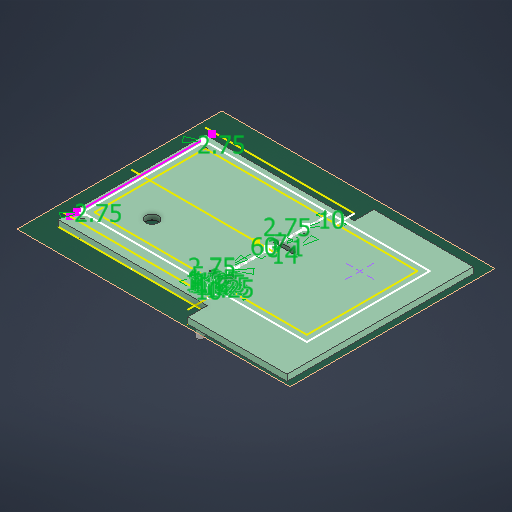
# Autodesk Inventor part: top-buggy-body-assembly-ready-group2
Saved by Autodesk Inventor 2026.2 (Build 302298010, 298A)
## iProperties
Created: 2026-02-09
Part Number: top-buggy-body-assembly-ready-group2
Material: Generic
Document SubType Name: Modeling
Designer: dm2166
Density: 1 g/cm^3
Appearance: Default
Mass: 226.605 g
Surface Area: 796.438 cm^2
Volume: 226.605 cm^3
Author: dm2166
Autodesk Inventor part; units mm, degrees
ref_plane "YZ Plane" through (0, 0, 0) normal (1, 0, 0) x (0, 1, 0)
ref_plane "XZ Plane" through (0, 0, 0) normal (0, 1, 0) x (-1, 0, 0)
ref_plane "XY Plane" through (0, 0, 0) normal (0, 0, 1) x (1, 0, 0)
sketch "Sketch1" plane through (0, 0, 0) normal (0, 1, 0) x (-1, 0, 0)
  line L0 (-85.5, -44.5) -> (85.5, -44.5)
  line L1 (85.5, -44.5) -> (85.5, 44.5)
  line L2 (85.5, 44.5) -> (-85.5, 44.5)
  line L3 (-85.5, 44.5) -> (-85.5, -44.5)
  line L4 (-85.5, -44.5) -> (85.5, 44.5) construction
  line L5 (85.5, -44.5) -> (-85.5, 44.5) construction
  line L6 (-81, -38.5) -> (81, -38.5)
  line L7 (81, -38.5) -> (81, 38.5)
  line L8 (81, 38.5) -> (-81, 38.5)
  line L9 (-81, 38.5) -> (-81, -38.5)
  line L10 (-81, -38.5) -> (81, 38.5) construction
  line L11 (81, -38.5) -> (-81, 38.5) construction
  line L12 (81, 38.5) -> (79.55, 38.5)
  line L13 (81, 37.05) -> (81, 38.5)
  circle A0 centre (79.55, 36.5) radius 1.45
  circle A1 centre (79.55, -36.5) radius 1.45
  circle A2 centre (-79.55, -38.5) radius 1.45
  circle A3 centre (-79.55, 38.4727) radius 1.45
  line L14 (81, -38.5) -> (81, -35.6)
  line L15 (-81, -38.5) -> (-78.1, -38.5)
  line L16 (-81, 38.5) -> (-81, 35.6)
  circle A4 centre (-79.55, 38.4727) radius 2.5
  line L17 (-95.5566, 0) -> (75.4434, 0)
  line L18 (0, 31.9167) -> (0, -57.0833)
  circle A5 centre (-79.55, -38.5) radius 2.5
  circle A6 centre (79.55, 36.5) radius 2.5
  circle A7 centre (79.55, -36.5) radius 2.5
  line L19 (140, 0) -> (-140, 0) projected
  line L20 (0, -105) -> (0, 105) projected
  line L21 (-100, 59.2475) -> (100, 59.2475)
  line L22 (100, 59.2475) -> (100, -59.2475)
  line L23 (100, -59.2475) -> (-100, -59.2475)
  line L24 (-100, -59.2475) -> (-100, 59.2475)
  line L25 (-100, 59.2475) -> (100, -59.2475) construction
  line L26 (100, 59.2475) -> (-100, -59.2475) construction
  line L27 (-100, 75) -> (-20, 75)
  line L28 (-20, 75) -> (-20, -75)
  line L29 (-20, -75) -> (-100, -75)
  line L30 (-100, -75) -> (-100, 75)
  line L31 (-100, 75) -> (-20, -75) construction
  line L32 (-20, 75) -> (-100, -75) construction
  line L33 (-79.55, 38.5) -> (-79.55, -38.5)
  line L34 (79.55, 36.5) -> (79.55, -36.5)
  line L35 (-96.0841, 75) -> (-26.0841, 75)
  line L36 (-26.0841, -75) -> (-94.0841, -75)
  point P0 (0, 0)
  point P1 (-80.9997, 38.5)
  point P2 (-81, 38.4727)
  point P3 (-81, -38.5)
  point P4 (-81, -38.5)
  point P5 (79.55, -38.5)
  point P6 (81, -36.5)
  point P7 (81, 36.5)
  point P8 (-60, 0)
  point P9 (-20, 59.2475)
  point P10 (-20, -59.2475)
  point P11 (-79.55, 0)
  point P12 (-78.1003, 38.5)
  point P13 (79.55, 0)
  dimension "d0" = 171
  dimension "d1" = 89
  dimension "d2" = 162
  dimension "d3" = 77
  dimension "d7" = 2.9
  dimension "d8" = 2.9
  dimension "d9" = 2.9
  dimension "d10" = 2.9
  dimension "d53" = 5
  dimension "d56" = 200
  dimension "d57" = 80
  dimension "d58" = 150
  dimension "d82" = 77
  dimension "d84" = 36.5
  dimension "d85" = 36.5
  constraints: 70 end point, 11 parallel, 10 midpoint, 8 centre point, 7 horizontal, 6 perpendicular, 5 point on line, 3 collinear, 3 concentric, 1 vertical, 4 other
  measures "d0" distance of L2.end L1.end
  measures "d1" distance of L1.end L0.end
  measures "d2" distance of L8.end L7.end
  measures "d3" distance of L7.end L6.end
  measures "d7" diameter of A0
  measures "d8" diameter of A1
  measures "d9" diameter of A2
  measures "d10" diameter of A3
  measures "d53" diameter of A4
  measures "d56" distance of L22.end L23.end
  measures "d57" distance of L28.end L29.end
  measures "d58" distance of L27.end L28.end
  measures "d82" distance of L33.start L33.end
  measures "d84" distance of point (79.55, 0) A1.centre
  measures "d85" distance from line of L19 A0.centre
extrude "Extrusion1" add sketch "Sketch1" along normal blind 55 contours A2 L6 | L6 L33 A2 | L8 L33 A3 | A3 L8 | A2 L33 L6 | L33 L8 A3 | A1 | A0
extrude "Extrusion2" add sketch "Sketch1" along normal blind 10 contours L28 L17 L18 L6 | L6 A5 L33 L17 L28 | L17 L33 A5 L9 | L9 A4 L33 L17 | L18 L17 L19 L34 A7 L6 | L6 A2 L33 A5 | L28 L8 L20 L18 L17 | L17 L33 A4 L8 L28 | A5 L33 A2 L9 | A7 L34 A1 L7 L6 | L18 L20 L8 A6 L34 L19 L17 | L6 L33 A2 | L8 L33 A3 | L9 A3 L33 A4 | A2 L33 L6 | L33 A3 L8 A4 | L19 L34 A6 L7 | L7 A7 L34 L19 | A7 L7 A1 L34 | L33 L8 A3 | A6 L34 A0 L7 | A1 | L8 L7 A0 L34 A6 | A0
extrude "Extrusion3" add sketch "Sketch1" along normal blind 25 contours L3 L17 L9 A5 L6 L28 L0 | L28 L6 L18 L0 | L3 L2 L28 L8 A4 L9 L17 | L18 L6 A7 L7 L19 L1 L0 | A5 L9 A2 L6 | L2 L20 L8 L28 | L19 L7 A6 L8 L20 L2 L1 | L6 L7 A7 | A2 L6 | A4 L8 A3 L9 | A3 L8 | L7 L8 A6
chamfer "Chamfer1" distance 2 angle 45 4 edges at (0, 25, 44.5) (85.5, 25, 0) (0, 25, -44.5) (-85.5, 25, 0)
extrude "Extrusion11" add sketch "Sketch1" along normal blind 45 contours A5 L9 A2 L6 | L6 A2 L33 A5 | A5 L33 A2 L9 | A7 L34 A1 L7 L6 | L6 L7 A7 | A2 L6 | L6 L33 A2 | L8 L33 A3 | A4 L8 A3 L9 | A3 L8 | L9 A3 L33 A4 | A2 L33 L6 | L33 A3 L8 A4 | A7 L7 A1 L34 | L33 L8 A3 | A6 L34 A0 L7 | L7 L8 A6 | A1 | L8 L7 A0 L34 A6 | A0
extrude "Extrusion12" add sketch "Sketch1" along normal blind 10 contours L0 L28 L23 L24 L19 L17 L3 | L0 L18 L20 L23 L28 | L17 L19 L24 L21 L28 L2 L3 | L0 L1 L19 L22 L23 L20 L18 | L28 L29 L30 L23 | L28 L21 L20 L2 | L1 L2 L20 L21 L22 L19 | L21 L30 L27 L28
chamfer "Chamfer2" distance 2 angle 45 8 edges at (100, 10, 0) (60, 10, 75) (20, 10, 67.1238) (60, 10, -75) (20, 10, -67.1238) (-40, 10, -59.2475) (-40, 10, 59.2475) (-100, 10, 0)
sketch "Sketch4" plane through (0, 0, 0) normal (0, -1, 0) x (1, 0, 0)
  circle A0 centre (-11.2675, 0) radius 2 projected
  circle A1 centre (-71.2675, 0) radius 2 projected
  circle A2 centre (-41.2675, 30) radius 2 projected
  circle A3 centre (-11.2675, 0) radius 2.5
  circle A4 centre (-71.2675, 0) radius 2.5
  circle A5 centre (-41.2675, 30) radius 2.5
  point P0 (0, 0)
  dimension "d64" = 5
  constraints: 3 centre point, 3 coincident, 2 equal radius
  measures "d64" diameter of A5
extrude "Extrusion13" add sketch "Sketch4" along normal blind 10 contours A0 | A1 | A2 | A3 | A4 | A5
sketch "Sketch7" plane through (0, 0, 0) normal (0, -1, 0) x (1, 0, 0)
  line L0 (20, -59.2475) -> (-100, -59.2475) projected
  line L1 (20, -75) -> (20, -59.2475) projected
  line L2 (100, -75) -> (20, -75) projected
  line L3 (100, 75) -> (100, -75) projected
  line L4 (20, 75) -> (100, 75) projected
  line L5 (20, 59.2475) -> (20, 75) projected
  line L6 (-100, 59.2475) -> (20, 59.2475) projected
  line L7 (-100, -59.2475) -> (-100, 59.2475) projected
  line L8 (-95, -54.2475) -> (25, -54.2475)
  line L9 (25, -54.2475) -> (25, -70)
  line L10 (25, -70) -> (95, -70)
  line L11 (95, -70) -> (95, 70)
  line L12 (95, 70) -> (25, 70)
  line L13 (25, 70) -> (25, 54.2475)
  line L14 (25, 54.2475) -> (-95, 54.2475)
  line L15 (-95, 54.2475) -> (-95, -54.2475)
  line L16 (-90, -49.2475) -> (30, -49.2475)
  line L17 (30, -49.2475) -> (30, -65)
  line L18 (30, -65) -> (90, -65)
  line L19 (90, -65) -> (90, 65)
  line L20 (90, 65) -> (30, 65)
  line L21 (30, 65) -> (30, 49.2475)
  line L22 (30, 49.2475) -> (-90, 49.2475)
  line L23 (-90, 49.2475) -> (-90, -49.2475)
  circle A0 centre (25, -70) radius 2.5
  circle A1 centre (25, 70) radius 2.5
  circle A2 centre (-41.2675, 0) radius 44 projected
  line L24 (-41.2675, -59.2475) -> (-41.2675, 59.2475)
  line L25 (17.4651, 0) -> (-100, 0)
  point P0 (0, 0)
  dimension "d86" = 5
  dimension "d87" = 10
  dimension "d88" = 5
  dimension "d89" = 5
  constraints: 36 end point, 3 midpoint, 2 centre point, 2 coincident, 1 perpendicular, 1 point on line, 14 other
  measures "d86" distance between parallel lines of L0 L8
  measures "d87" distance between parallel lines of L0 L16
  measures "d88" diameter of A0
  measures "d89" diameter of A1
extrude "Extrusion15" add sketch "Sketch7" along normal blind 10 contours A0 L10 L9 | L9 L10 A0 | A1 L12 L13 | L13 L12 A1
fillet "Fillet16" radius 1 1 edges at (22.5, -10, -70)
fillet "Fillet17" radius 1 1 edges at (22.5, 0, -70)
fillet "Fillet18" radius 1 1 edges at (22.5, 0, 70)
fillet "Fillet19" radius 1 1 edges at (22.5, -10, 70)
sketch "Sketch9" plane through (0, 0, 0) normal (0, -1, 0) x (1, 0, 0)
  line L0 (-100, 59.2475) -> (20, 59.2475) projected
  line L1 (20, -75) -> (20, 75) projected
  line L2 (20, -59.2475) -> (-100, -59.2475) projected
  line L3 (-100, -59.2475) -> (-100, 59.2475) projected
  circle A0 centre (-41.2675, 0) radius 44 projected
  line L4 (-41.2675, -59.2475) -> (-41.2675, 59.2475)
  line L5 (17.4651, 0) -> (-100, 0)
  line L6 (20, -54.2475) -> (-95, -54.2475)
  line L7 (-95, -54.2475) -> (-95, 54.2475)
  line L8 (-95, 54.2475) -> (20, 54.2475)
  line L9 (-41.2675, 50.5475) -> (-41.2675, 47.5475)
  point P0 (0, 0)
  point P1 (-41.2675, -54.2475)
  point P2 (-41.2675, 54.2475)
  constraints: 12 end point, 4 point on line, 3 midpoint, 1 perpendicular, 1 symmetric about line, 2 other
sketch "Sketch11" plane through (0, 10, 0) normal (0, 1, 0) x (1, 0, 0)
  circle A0 centre (-168.2379, -151.522) radius 7.5
  circle A1 centre (-62.4807, -21.2132) radius 7.5 projected
  circle A2 centre (-62.4807, -21.2132) radius 5
  point P0 (0, 0)
  dimension "d134" = 10
  constraints: 2 centre point, 1 coincident
  measures "d134" diameter of A2
sketch "Sketch12" plane through (0, 10, 0) normal (0, 1, 0) x (1, 0, 0)
  line L0 (-85.5, -44.5) -> (85.5, -44.5) projected
  line L1 (-85.5, 44.5) -> (-85.5, -44.5) projected
  line L2 (85.5, 44.5) -> (-85.5, 44.5) projected
  line L3 (85.5, -44.5) -> (85.5, 44.5) projected
  line L4 (90.5, -49.5) -> (-90.5, -49.5)
  line L5 (-90.5, -49.5) -> (-90.5, 49.5)
  line L6 (-90.5, 49.5) -> (90.5, 49.5)
  line L7 (90.5, 49.5) -> (90.5, -49.5)
  circle A0 centre (-90.5, 49.5) radius 1.375
  circle A1 centre (-90.5, -49.5) radius 1.375
  line L8 (20, -59.2475) -> (20, -75) projected
  line L9 (20, -59.2475) -> (20, -44.5)
  line L10 (20, 59.2475) -> (-100, 59.2475) projected
  line L11 (20, 59.2475) -> (20, 44.5)
  line L12 (20, -49.5) -> (10, -49.5)
  line L13 (20, 49.5) -> (10, 49.5)
  line L14 (17.4651, 0) -> (-100, 0) projected
  line L15 (10, 49.5) -> (10, -49.5)
  line L16 (10, 30) -> (10, -30)
  circle A2 centre (10, -30) radius 1.375
  circle A3 centre (10, 30) radius 1.375
  point P0 (0, 0)
  point P1 (62.481, 21.213)
  point P2 (10, 0)
  dimension "d120" = 5
  dimension "d123" = 2.75
  dimension "d124" = 2.75
  dimension "d127" = 10
  dimension "d128" = 10
  dimension "d162" = 60
  dimension "d163" = 2.75
  dimension "d164" = 2.75
  constraints: 20 end point, 10 point on line, 6 coincident, 4 centre point, 2 midpoint, 1 perpendicular, 3 other
  measures "d120" distance between parallel lines of L0 L4
  measures "d123" diameter of A0
  measures "d124" diameter of A1
  measures "d127" distance of L12.start L12.end
  measures "d128" distance of L13.start L13.end
  measures "d162" distance of L16.start L16.end
  measures "d163" diameter of A2
  measures "d164" diameter of A3
extrude "Extrusion19" cut sketch "Sketch12" against normal blind 14 contours A1 L5 L4 | L4 L5 A1 | A0 L6 L5 | L5 L6 A0
extrude "Extrusion20" [suppressed]
fillet "Fillet21" radius 1 6 edges at (-73.7675, 0, 0) (-73.7675, -10, 0) (-43.7675, -10, 30) (-43.7675, 0, 30) (-13.7675, 0, 0) (-13.7675, -10, 0)
extrude "Extrusion21" cut sketch "Sketch11" against normal blind 14 contours A2
fillet "Fillet22" radius 1 2 edges at (-67.4807, 0, 21.2132) (-67.4807, 10, 21.2132)
sketch "Sketch13" plane through (0, 0, 0) normal (0, -1, 0) x (1, 0, 0)
  line L0 (-95, 54.2475) -> (20, 54.2475) projected
  line L1 (6.8242, 54.2475) -> (3.8242, 54.2475)
  point P0 (0, 0)
  point P1 (11.8242, 54.2475)
  point P2 (-21.0705, 54.2475)
  constraints: 3 point on line, 2 end point
sketch "Sketch14" plane through (0, 10, 0) normal (0, 1, 0) x (1, 0, 0)
  line L0 (-98, 57.2475) -> (22, 57.2475) projected
  line L1 (-98, -57.2475) -> (-98, 57.2475) projected
  line L2 (22, -57.2475) -> (-98, -57.2475) projected
  line L3 (-85.5, -44.5) -> (85.5, -44.5) projected
  line L4 (-85.5, 44.5) -> (-85.5, -44.5) projected
  line L5 (85.5, 44.5) -> (-85.5, 44.5) projected
  line L6 (85.5, -44.5) -> (85.5, 44.5) projected
  line L7 (98, 73) -> (98, -73) projected
  line L8 (100, 75) -> (20, 75) projected
  line L9 (22, 57.2475) -> (22, 73) projected
  line L10 (22, 73) -> (98, 73) projected
  line L11 (98, -73) -> (22, -73) projected
  line L12 (22, -73) -> (22, -57.2475) projected
  point P0 (0, 0)
extrude "Extrusion22" add sketch "Sketch14" along normal blind 10
ref_plane "Work Plane3" through (0, 20, 0) normal (0, 1, 0) x (1, 0, 0)
sketch "Sketch17" plane through (0, 10, 0) normal (0, 1, 0) x (1, 0, 0)
  line L0 (-92.5566, -57.2475) -> (-92.5566, 57.2475) projected
  line L1 (-98, -57.2475) -> (22, -57.2475) projected
  point P0 (0, 0)
  point P1 (-92.5566, -51.8042)
extrude "Extrusion26" cut sketch "Sketch12" against normal through all contours A2 L15 | L15 A2 | A3 L15 | L15 A3
sketch "Sketch19" plane through (0, 20, 0) normal (0, 1, 0) x (1, 0, 0)
  line L0 (22, 57.2475) -> (-98, 57.2475) projected
  line L1 (22, 57.2475) -> (22, 44.5)
  line L2 (85.5, 44.5) -> (-85.5, 44.5) projected
  line L3 (22, 73) -> (22, 57.2475) projected
  line L4 (98, 73) -> (22, 73) projected
  line L5 (98, -73) -> (98, 73) projected
  line L6 (22, -73) -> (98, -73) projected
  line L7 (22, -57.2475) -> (22, -73) projected
  line L8 (-85.5, -44.5) -> (85.5, -44.5) projected
  line L9 (85.5, -44.5) -> (85.5, 44.5) projected
  line L10 (22, 57.2475) -> (22, 73) projected
  line L11 (22, 57.2475) -> (22, 73)
  line L12 (22, 73) -> (98, 73)
  line L13 (98, -73) -> (100, -75) projected
  line L14 (98, 73) -> (98, -73)
  line L15 (98, -73) -> (22, -73)
  line L16 (22, -73) -> (20, -75) projected
  line L17 (22, -57.2475) -> (22, -73)
  line L18 (22, -44.5) -> (85.5, -44.5)
  line L19 (85.5, -44.5) -> (85.5, 44.5)
  line L20 (85.5, 44.5) -> (22, 44.5)
  line L21 (22, -73) -> (98, -73)
  line L22 (-98, -57.2475) -> (22, -57.2475) projected
  line L23 (22, -57.2475) -> (22, -44.5)
  point P0 (0, 0)
  point P1 (22, -44.5)
  constraints: 22 end point, 4 collinear, 3 point on line, 3 vertical, 2 perpendicular
extrude "Extrusion27" cut sketch "Sketch19" against normal blind 10
sketch "Sketch20" plane through (22, 10, 57.2475) normal (1, 0, 0) x (0, 0, -1)
  line L0 (-0.0001, 10) -> (2.4999, 10)
  line L1 (0, 10) -> (12.7547, 10) projected
  line L2 (0, 0) -> (12.7475, 0) projected
  line L3 (2.4999, 10) -> (12.4999, 10)
  line L4 (12.4999, 10) -> (12.4999, 0)
  line L5 (12.4999, 0) -> (2.4999, 0)
  line L6 (2.4999, 0) -> (2.4999, 10)
  line L7 (12.4999, 10) -> (7.4999, 10)
  line L8 (7.4999, 10) -> (7.4999, 5)
  line L9 (7.4999, 5) -> (12.4999, 5)
  line L10 (12.4999, 5) -> (12.4999, 10)
  point P0 (57.2475, -10)
  point P1 (2.4999, 0)
  dimension "d170" = 2.5
  dimension "d171" = 10
  dimension "d172" = 5
  dimension "d173" = 5
  constraints: 18 end point, 4 parallel, 2 horizontal, 2 perpendicular, 2 point on line
  measures "d170" distance of L0.start L0.end
  measures "d171" distance of L4.end L5.end
  measures "d172" distance of L9.end L8.end
  measures "d173" distance of L8.end L7.end
extrude "Extrusion28" cut sketch "Sketch20" against normal through all contours L1 L8 L9 L4 L2 L6
sketch "Sketch21" plane through (-98, 10, 57.2475) normal (0, 0, 1) x (1, 0, 0)
  line L0 (0.0014, 10.0004) -> (2.5014, 10.0004)
  line L1 (0.0016, 10.0004) -> (12.7563, 10.0004)
  line L2 (0.0016, 0.0004) -> (12.7491, 0.0004)
  line L3 (2.5014, 10.0004) -> (12.5014, 10.0004)
  line L4 (12.5014, 10.0004) -> (12.5014, 0.0004)
  line L5 (12.5014, 0.0004) -> (2.5014, 0.0004)
  line L6 (2.5014, 0.0004) -> (2.5014, 10.0004)
  line L7 (12.5014, 10.0004) -> (7.5014, 10.0004)
  line L8 (7.5014, 10.0004) -> (7.5014, 5.0004)
  line L9 (7.5014, 5.0004) -> (12.5014, 5.0004)
  line L10 (12.5014, 5.0004) -> (12.5014, 10.0004)
  point P0 (98, -10)
  point P1 (40.8323, -6.0448)
  point P2 (-3.9153, 8.9552)
  point P3 (-8.9153, 13.9552)
  point P4 (-13.9153, 3.9552)
  point P5 (12.5014, 5.0004)
  point P6 (7.5014, 10.0004)
  point P7 (2.5014, 0.0004)
  dimension "d176" = 2.5
  dimension "d177" = 10
  dimension "d178" = 5
  dimension "d179" = 5
  constraints: 22 end point, 4 parallel, 2 horizontal, 2 perpendicular, 2 point on line
  measures "d176" distance of L0.start L0.end
  measures "d177" distance of L4.end L5.end
  measures "d178" distance of L9.end L8.end
  measures "d179" distance of L8.end L7.end
extrude "Extrusion29" cut sketch "Sketch21" against normal through all contours L1 L8 L9 L4 L2 L6
sketch "Sketch22" plane through (22, 20, -44.5) normal (1, 0, 0) x (0, 0, -1)
  line L0 (7.7461, 0.0193) -> (10.2461, 0.0193)
  line L1 (10.2461, -9.9807) -> (10.2461, 0.0193)
  line L2 (12.7461, 0.0193) -> (10.2461, 0.0193)
  line L3 (12.746, 0.0193) -> (-0.0087, 0.0193)
  line L4 (12.746, -9.9807) -> (-0.0015, -9.9807)
  line L5 (10.2461, 0.0193) -> (0.2461, 0.0193)
  line L6 (0.2461, 0.0193) -> (0.2461, -9.9807)
  line L7 (0.2461, -9.9807) -> (10.2461, -9.9807)
  line L8 (0.2461, 0.0193) -> (5.2461, 0.0193)
  line L9 (5.2461, 0.0193) -> (5.2461, -4.9807)
  line L10 (5.2461, -4.9807) -> (0.2461, -4.9807)
  line L11 (0.2461, -4.9807) -> (0.2461, 0.0193)
  point P0 (-44.5, -20)
  point P1 (44.663, -8.7349)
  point P2 (-0.0847, 6.2651)
  point P3 (-5.0847, 11.2651)
  point P4 (-10.0847, 1.2651)
  point P5 (0.2461, -4.9807)
  point P6 (10.2461, -9.9807)
  point P7 (5.2461, 0.0193)
  dimension "d186" = 2.5
  constraints: 24 end point, 2 point on line, 1 symmetric about line
  measures "d186" distance of L2.start L0.end
extrude "Extrusion30" cut sketch "Sketch22" against normal through all contours L0 L1 L4 L6 L10 L9 L3
sketch "Sketch23" plane through (0, 20, 0) normal (0, 1, 0) x (1, 0, 0)
  line L0 (-98, 54.7461) -> (-95.4986, 54.7461) projected
  line L1 (-98, 57.2475) -> (-98, 54.7461) projected
  line L2 (-95.4986, 54.7461) -> (-95.4986, 57.2475) projected
  line L3 (-95.4986, 57.2475) -> (-98, 57.2475) projected
  point P0 (0, 0)
extrude "Extrusion31" cut sketch "Sketch23" against normal blind 10
sketch "Sketch24" plane through (0, 20, 0) normal (0, 1, 0) x (1, 0, 0)
  line L0 (-98, -54.7476) -> (-98, -57.2475) projected
  line L1 (-98, -57.2475) -> (-95.4986, -57.2475) projected
  line L2 (-95.4986, -54.7476) -> (-98, -54.7476) projected
  line L3 (-95.4986, -57.2475) -> (-95.4986, -54.7476) projected
  point P0 (0, 0)
extrude "Extrusion32" cut sketch "Sketch24" against normal blind 10
sketch "Sketch25" plane through (0, 20, 0) normal (0, 1, 0) x (1, 0, 0)
  line L0 (-90.4986, 54.7461) -> (22, 54.7461) projected
  line L1 (22, 57.2475) -> (-90.4986, 57.2475) projected
  line L2 (-90.4986, 57.2475) -> (-90.4986, 54.7461) projected
  line L3 (-85.4986, 44.7461) -> (-85.4986, 54.7461) projected
  line L4 (-85.4986, -44.7476) -> (-85.4986, 57.2475) projected
  line L5 (-85.4986, 54.7461) -> (-85.4986, 57.2475)
  line L6 (-95.4986, 44.7461) -> (-98, 44.7461) projected
  line L7 (-98, 49.7461) -> (-98, -49.7476) projected
  line L8 (-95.4986, -49.7476) -> (-95.4986, 49.7461) projected
  line L9 (-95.4986, 49.7461) -> (-98, 49.7461) projected
  line L10 (-85.4986, -44.7476) -> (-95.4986, -44.7476) projected
  line L11 (-98, -49.7476) -> (-95.4986, -49.7476) projected
  line L12 (-95.4986, -44.7476) -> (-98, -44.7476)
  line L13 (-85.4986, -57.2475) -> (-85.4986, -54.7476) projected
  line L14 (22, -54.7476) -> (-90.4986, -54.7476) projected
  line L15 (-90.4986, -57.2475) -> (22, -57.2475) projected
  line L16 (-90.4986, -54.7476) -> (-90.4986, -57.2475) projected
  point P0 (0, 0)
  constraints: 4 end point, 2 point on line, 1 collinear
extrude "Extrusion33" cut sketch "Sketch25" against normal blind 10 contours L2 L1 L4 L0 | L6 L7 L9 L8 | L8 L11 L7 L12 | L15 L16 L14 L13
sketch "Sketch26" plane through (0, 0, 0) normal (0, -1, 0) x (1, 0, 0)
  line L0 (20, -75) -> (20, 75) projected
  line L1 (17.4651, 0) -> (-100, 0) projected
  line L2 (20, 0) -> (12.9841, 0)
  line L3 (12.9841, -28.85) -> (12.9841, 28.85)
  line L4 (12.9841, 28.85) -> (-4.0004, 28.85)
  line L5 (-4.0004, 28.85) -> (-4.0004, 39)
  line L6 (-4.0004, 39) -> (12.9841, 39)
  line L7 (12.9841, 39) -> (12.9841, 28.85)
  line L8 (12.9841, 28.85) -> (6.065, 28.85)
  line L9 (6.065, 28.85) -> (6.065, 39)
  line L10 (6.065, 39) -> (0.8687, 39)
  line L11 (0.8687, 39) -> (0.8687, 28.85)
  line L12 (-5.5234, 27.327) -> (14.5071, 27.327)
  line L13 (14.5071, 27.327) -> (14.5071, 40.523)
  line L14 (14.5071, 40.523) -> (-5.5234, 40.523)
  line L15 (-5.5234, 40.523) -> (-5.5234, 27.327)
  line L16 (12.9841, 33.925) -> (-4.0004, 33.925)
  line L17 (9.5246, 28.85) -> (9.5246, 39)
  line L18 (4.4918, 28.85) -> (3.4668, 39)
  line L19 (-1.5, 39) -> (-1.5, 28.85)
  line L20 (12.9841, 33.925) -> (11.7341, 33.925)
  line L21 (9.5246, 33.925) -> (8.2746, 33.925)
  line L22 (6.065, 33.925) -> (4.815, 33.925)
  line L23 (3.9793, 33.925) -> (2.7293, 33.925)
  line L24 (0.8687, 33.925) -> (-0.3813, 33.925)
  line L25 (-1.5, 33.925) -> (-2.75, 33.925)
  circle A0 centre (11.7341, 33.925) radius 0.75
  circle A1 centre (8.2746, 33.925) radius 0.75
  circle A2 centre (4.815, 33.925) radius 0.75
  circle A3 centre (2.7293, 33.925) radius 0.75
  circle A4 centre (-0.3813, 33.925) radius 0.75
  circle A5 centre (-2.75, 33.925) radius 0.75
  line L26 (17.7288, -22.3769) -> (17.7288, -15.3769)
  line L27 (17.7288, -15.3769) -> (3.7288, -15.3769)
  line L28 (3.7288, -15.3769) -> (3.7288, -22.3769)
  line L29 (3.7288, -22.3769) -> (17.7288, -22.3769)
  line L30 (22, -54.7461) -> (-85.4986, -54.7461) projected
  line L31 (17.7288, -22.3769) -> (3.7288, -15.3769) construction
  line L32 (17.7288, -15.3769) -> (3.7288, -22.3769) construction
  line L33 (18.7288, -23.3769) -> (18.7288, -14.3769)
  line L34 (18.7288, -14.3769) -> (2.7288, -14.3769)
  line L35 (2.7288, -14.3769) -> (2.7288, -23.3769)
  line L36 (2.7288, -23.3769) -> (18.7288, -23.3769)
  line L37 (18.7288, -14.3769) -> (2.7288, -14.3769)
  line L38 (2.7288, -14.3769) -> (2.7288, -11.3769)
  line L39 (2.7288, -11.3769) -> (18.7288, -11.3769)
  line L40 (18.7288, -11.3769) -> (18.7288, -14.3769)
  line L41 (3.7288, -22.3769) -> (3.7288, -23.3769)
  line L42 (3.7288, -15.3769) -> (2.7288, -15.3769)
  line L43 (3.7288, -22.3769) -> (2.7288, -22.3769)
  line L44 (17.7288, -22.3769) -> (18.7288, -22.3769)
  line L45 (17.7288, -15.3769) -> (18.7288, -15.3769)
  point P0 (0, 0)
  point P1 (10.7288, -18.8769)
  dimension "d220" = 1.25
  dimension "d221" = 1.25
  dimension "d222" = 1.25
  dimension "d223" = 1.25
  dimension "d224" = 1.25
  dimension "d225" = 1.25
  dimension "d226" = 1.5
  dimension "d227" = 1.5
  dimension "d228" = 1.5
  dimension "d229" = 1.5
  dimension "d230" = 1.5
  dimension "d231" = 1.5
  dimension "d240" = 7
  dimension "d241" = 14
  dimension "d254" = 1
  dimension "d255" = 3
  constraints: 84 end point, 14 midpoint, 14 point on line, 10 parallel, 10 perpendicular, 6 centre point, 6 coincident, 3 vertical, 2 horizontal, 1 collinear, 17 other
  measures "d220" distance of L20.start L20.end
  measures "d221" distance of L21.start L21.end
  measures "d222" distance of L22.start L22.end
  measures "d223" distance of L23.start L23.end
  measures "d224" distance of L24.start L24.end
  measures "d225" distance of L25.start L25.end
  measures "d226" diameter of A0
  measures "d227" diameter of A1
  measures "d228" diameter of A2
  measures "d229" diameter of A3
  measures "d230" diameter of A4
  measures "d231" diameter of A5
  measures "d240" distance of L28.end L27.end
  measures "d241" distance of L27.end L26.end
  measures "d254" distance between parallel lines of L29 L36
  measures "d255" distance of L37.end L38.end
extrude "Extrusion36" cut sketch "Sketch26" against normal through all contours A0 L16 | L16 A0 | A1 L16 | L16 A1 | A2 L16 | L16 A2 | A3 L16 | L16 A3 | A4 L16 | L16 A4 | A5 L16 | L16 A5
extrude "Extrusion37" add sketch "Sketch26" along normal blind 5 contours L15 L14 L13 L12
fillet "Fillet24" radius 0.5 4 edges at (-5.5234, -5, 33.925) (4.4918, -5, 27.327) (14.5071, -5, 33.925) (4.4918, -5, 40.523)
fillet "Fillet25" radius 0.5 3 edges at (-38, 10, 44.7476) (-31.7493, 10, 54.7476) (-31.7493, 15, 49.7476)
fillet "Fillet26" radius 0.5 2 edges at (-95.4986, 10.0004, 0.2407) (-90.4986, 15.0004, 2.5008)
fillet "Fillet27" radius 0.5 3 edges at (-31.7493, 10.0193, -44.7461) (-31.7493, 10.0193, -54.7461) (-34.0676, 15.0193, -49.7461)
sketch "Sketch27" plane through (0, 0, 0) normal (0, -1, 0) x (1, 0, 0)
  point P0 (0, 0)
extrude "Extrusion40" add sketch "Sketch26" along normal blind 3 contours L43 L35 L42 L28 | L26 L45 L33 L44
extrude "Extrusion41" cut sketch "Sketch26" against normal through all contours L34 L38 L39 L3 | L3 L39 L40 L34
chamfer "Chamfer7" distance 0.3 angle 45 4 edges at (17.7288, -1.5, -15.3769) (3.7288, -1.5, -15.3769) (17.7288, -1.5, -22.3769) (3.7288, -1.5, -22.3769)
ref_plane "Work Plane5" through (0, 5, 0) normal (0, -1, 0) x (1, 0, 0)
split "Split1" plane through (0, 5, 0) removes the side toward (0, 1, 0)
body "Solid1"
